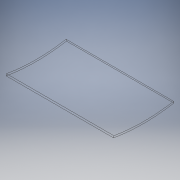
# Autodesk Inventor part: element_3
Saved by Autodesk Inventor 2018.1 (Build 221171000, 171)
## iProperties
Created: 2017-10-18
Part Number: element_3
Material: CFRP
Document SubType Name: Modeling
Designer: kuwano
Density: 1.43 g/cm^3
Appearance: カーボンファイバー
Mass: 108.358 g
Surface Area: 526.228 cm^2
Volume: 75.7748 cm^3
Author: kuwano
Autodesk Inventor part; units mm, degrees
ref_plane "YZ Plane" through (0, 0, 0) normal (1, 0, 0) x (0, 1, 0)
ref_plane "XZ Plane" through (0, 0, 0) normal (0, 1, 0) x (-1, 0, 0)
ref_plane "XY Plane" through (0, 0, 0) normal (0, 0, 1) x (1, 0, 0)
sketch "スケッチ1" plane through (0, 0, 0) normal (1, 0, 0) x (0, 1, 0)
  arc A0 (7.3744, 50) -> (7.3744, -50) centre (290.9385, 0) ccw
  arc A1 (4.42, 50.5209) -> (4.42, -50.5209) centre (290.9385, 0) ccw
  line L0 (7.3744, 50) -> (4.42, 50.5209)
  line L1 (7.3744, -50) -> (4.42, -50.5209)
  line L2 (0, -70.7293) -> (0, 70.7293) projected
  point P0 (0, 0)
  point P1 (0, 0)
  dimension "d0" = 3
  dimension "d1" = 100
  dimension "d2" = 20
  constraints: 5 point on circle, 4 end point, 4 line through centre, 2 centre point, 1 coincident, 1 concentric, 1 tangent
  measures "d0" distance of L0.start L0.end
  measures "d1" distance of L1.start L0.start
  measures "d2" angle of L1 L0
extrude "押し出し1" add sketch "スケッチ1" along normal blind 250
